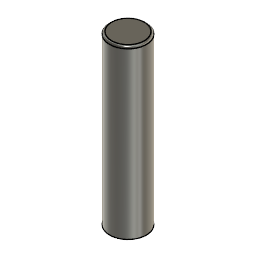
GuideRod (Autodesk Fusion 360 design; units mm, degrees)
part number: 2026-05-26-20-31-48-978
Autodesk Fusion 360 part; units mm, degrees
sketch "Sketch3" plane through (0, 0, 0) normal (0, 0, 1) x (1, 0, 0)
  circle A0 centre (0, 0) radius 4.4
  dimension "d4" = 8.8
  constraint coincident A0.centre origin
  measures "d4" diameter of A0
extrude "Extrude1" add sketch "Sketch3" along normal blind 40
fillet "Fillet1" radius 0.5 1 edges at (-4.1022, -1.5911, 40)
equation "Tolerance = 0.1 mm"
equation "d4 = 9 mm - 2 * Tolerance"
